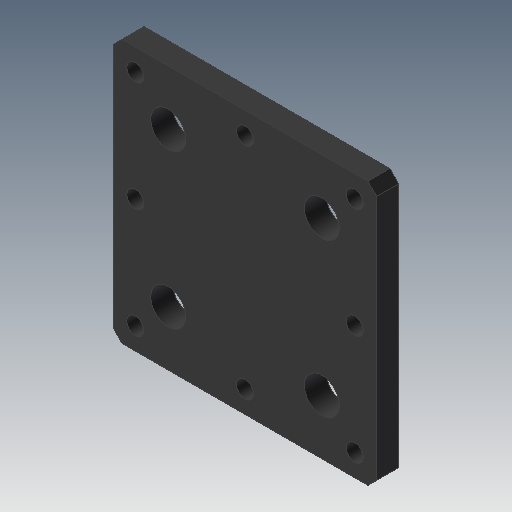
# Autodesk Inventor part: cellSTORM_v5_spacer_xy_stage
Saved by Autodesk Inventor 2019.4 (Build 234330000, 330)
## iProperties
Created: 2020-07-01
Part Number: cellSTORM_v5_spacer_xy_stage
Material: Generic
Document SubType Name: Modeling
Designer: diederichbenedict
Density: 1 g/cm^3
Appearance: Default
Author: diederichbenedict
Autodesk Inventor part; units mm, degrees
ref_plane "YZ Plane" through (0, 0, 0) normal (1, 0, 0) x (0, 1, 0)
ref_plane "XZ Plane" through (0, 0, 0) normal (0, 1, 0) x (-1, 0, 0)
ref_plane "XY Plane" through (0, 0, 0) normal (0, 0, 1) x (1, 0, 0)
sketch "Sketch1" plane through (0, 0, 0) normal (0, 0, 1) x (1, 0, 0)
  line L0 (100.1576, -44) -> (109, -35.1576) projected
  line L1 (109, -35.1576) -> (109, 35) projected
  line L2 (109, 35) -> (41.05, 35) projected
  line L3 (41.05, 35) -> (28, 30) projected
  line L4 (28, 30) -> (-28, 30) projected
  line L5 (-28, 30) -> (-30, 28) projected
  line L6 (-30, 28) -> (-30, -28) projected
  line L7 (-30, -28) -> (-28, -30) projected
  line L8 (-28, -30) -> (28, -30) projected
  line L9 (28, -30) -> (90.0667, -30) projected
  line L10 (90.0667, -30) -> (90.0667, -44) projected
  line L11 (90.0667, -44) -> (100.1576, -44) projected
  circle A0 centre (101, -8.23) radius 1.6 projected
  circle A1 centre (101, 1.77) radius 1.6 projected
  circle A2 centre (101, 29.77) radius 1.6 projected
  circle A3 centre (85, 29.77) radius 1.6 projected
  circle A4 centre (85, 1.77) radius 1.6 projected
  circle A5 centre (85, -8.23) radius 1.6 projected
  circle A6 centre (64.15, 11.27) radius 1.6 projected
  circle A7 centre (47.85, 11.27) radius 1.6 projected
  circle A8 centre (25, 0) radius 1.95 projected
  circle A9 centre (0, 25) radius 1.95 projected
  circle A10 centre (-25, -25) radius 1.95 projected
  circle A11 centre (25, 25) radius 1.95 projected
  circle A12 centre (-25, 25) radius 1.95 projected
  circle A13 centre (25, -25) radius 1.95 projected
  circle A14 centre (0, -25) radius 1.95 projected
  circle A15 centre (-25, 0) radius 1.95 projected
  circle A16 centre (-17.5, 17.5) radius 4 projected
  circle A17 centre (17.5, -17.5) radius 4 projected
  circle A18 centre (-17.5, -17.5) radius 4 projected
  circle A19 centre (17.5, 17.5) radius 4 projected
  line L12 (30, 28) -> (28, 30) projected
  line L13 (30, -28) -> (30, 28) projected
  line L14 (28, -30) -> (30, -28) projected
  point P0 (0, 0)
extrude "Extrusion1" add sketch "Sketch1" along normal blind 5 contours L8 L7 L6 L5 L4 L12 L13 L14
body "Solid1"
